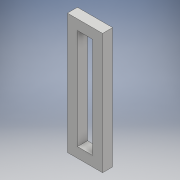
# Autodesk Inventor part: Palm_Hand_Velcro_Strap_Buckle_(Version_1)
Saved by Autodesk Inventor 2017 (Build 210142000, 142)
## iProperties
Created: 2019-11-25
Part Number: Palm_Hand_Velcro_Strap_Buckle_(Version_1)
Material: Generic
Document SubType Name: Modeling
Designer: asadb
Density: 1 g/cm^3
Appearance: Default
Author: asadb
Autodesk Inventor part; units mm, degrees
ref_plane "YZ Plane" through (0, 0, 0) normal (1, 0, 0) x (0, 1, 0)
ref_plane "XZ Plane" through (0, 0, 0) normal (0, 1, 0) x (-1, 0, 0)
ref_plane "XY Plane" through (0, 0, 0) normal (0, 0, 1) x (1, 0, 0)
sketch "Sketch1" plane through (0, 0, 0) normal (0, 1, 0) x (-1, 0, 0)
  line L0 (0, 0) -> (3, 0)
  line L1 (3, 0) -> (3, -20)
  line L2 (3, -20) -> (0, -20)
  line L3 (0, -20) -> (0, 0)
  line L4 (5, -22) -> (5, 2)
  line L5 (5, 2) -> (-2, 2)
  line L6 (-2, 2) -> (-2, -22)
  line L7 (-2, -22) -> (5, -22)
  dimension "d0" = 3
  dimension "d1" = 20
  dimension "d2" = 2
  constraints: 16 end point, 4 parallel, 2 perpendicular, 1 horizontal, 3 other
  measures "d0" distance of L1.end L2.end
  measures "d1" distance of L0.end L1.end
  measures "d2" distance between parallel lines of L1 L4
extrude "Extrusion1" add sketch "Sketch1" along normal blind 2
body "Solid1"
